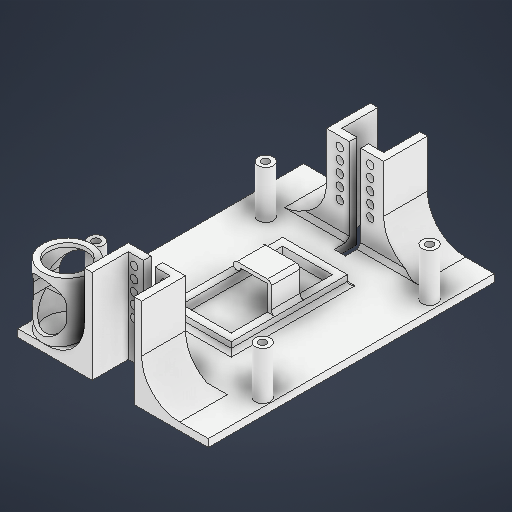
# Autodesk Inventor part: CHASIS
Saved by Autodesk Inventor 2027 (Build 310192060, 192F)
## iProperties
Created: 2026-05-31
Part Number: CHASIS
Material: Genérico
Document SubType Name: Modeling
Designer: noemi
Density: 1 g/cm^3
Appearance: Valor por defecto
Author: noemi
Autodesk Inventor part; units mm, degrees
ref_plane "YZ Plane" through (0, 0, 0) normal (1, 0, 0) x (0, 1, 0)
sketch "Boceto1" plane through (0, 0, 0) normal (0, 1, 0) x (-1, 0, 0)
  line L0 (0, 0) -> (100, 0)
  line L1 (100, 0) -> (100, -150)
  line L2 (100, -150) -> (0, -150)
  line L3 (0, -150) -> (0, 0)
  dimension "d0" = 150
  dimension "d1" = 100
  constraints: 8 end point, 3 perpendicular, 1 horizontal
  measures "d0" distance of L0.end L1.end
  measures "d1" distance of L1.end L2.end
extrude "Extrusión1" add sketch "Boceto1" along normal blind 4
sketch "Boceto2" plane through (0, 4, 0) normal (0, 1, 0) x (1, 0, 0)
  line L0 (-100, 0) -> (0, 0) projected
  line L1 (0, 0) -> (0, 150) projected
  line L2 (-100, 0) -> (0, 0)
  line L3 (-50, 0) -> (-50, 19)
  line L4 (-61, 0) -> (-61, 19)
  line L5 (-39, 0) -> (-39, 19)
  line L6 (-61, 19) -> (-39, 19)
  line L7 (0, 75) -> (-100, 75)
  line L8 (-65, 0) -> (-65, 23)
  line L9 (-65, 23) -> (-35, 23)
  line L10 (-35, 23) -> (-35, 0)
  line L11 (-100, 150) -> (0, 150)
  line L12 (-61, 150) -> (-61, 131)
  line L13 (-39, 150) -> (-39, 131)
  line L14 (-61, 131) -> (-39, 131)
  line L15 (-65, 150) -> (-65, 127)
  line L16 (-65, 127) -> (-35, 127)
  line L17 (-35, 127) -> (-35, 150)
  dimension "d4" = 19
  dimension "d5" = 11
  dimension "d6" = 11
  dimension "d7" = 19
  dimension "d8" = 0
  dimension "d9" = 0
  dimension "d10" = 100
  dimension "d11" = 4
  constraints: 32 end point, 9 symmetric about line, 2 horizontal, 2 midpoint, 2 parallel, 1 perpendicular, 1 vertical, 2 other
  measures "d4" distance of L3.start L3.end
  measures "d5" distance between parallel lines of L3 L4
  measures "d6" distance between parallel lines of L3 L5
  measures "d7" distance between parallel lines of L6 L0
  measures "d8" distance from line of L5.start L0
  measures "d9" distance from line of L4.start L0
  measures "d10" distance from line of L7.end L1
  measures "d11" distance between parallel lines of L4 L8
extrude "Extrusión2" cut sketch "Boceto2" against normal blind 4 contours L4 L6 L3 L0 | L3 L6 L5 L0 | L13 L14 L12 L11
extrude "Extrusión3" add sketch "Boceto2" along normal blind 45 contours L8 L9 L10 L0 L5 L6 L4 | L17 L16 L15 L11 L12 L14 L13
sketch "Boceto3" plane through (-61, 0, -19) normal (0, 0, 1) x (1, 0, 0)
  circle A0 centre (3, 44) radius 2
  line L0 (0, 49) -> (22, 49) projected
  line L1 (11, 49) -> (11, 33.933)
  circle A1 centre (19, 44) radius 2
  point P0 (61, 0)
  dimension "d16" = 4
  dimension "d17" = 8
  dimension "d25" = 5
  constraints: 2 centre point, 2 end point, 1 midpoint, 1 perpendicular, 1 symmetric about line, 1 other
  measures "d16" diameter of A0
  measures "d17" distance from line of L1 A0.centre
  measures "d25" distance from line of L0 A0.centre
extrude "Extrusión4" cut sketch "Boceto3" against normal up to surface (112 mm away)
sketch "Boceto4" plane through (0, 0, 0) normal (0, -1, 0) x (1, 0, 0)
  line L0 (-61, -150) -> (-61, -131) projected
  line L1 (-61, -131) -> (-39, -131) projected
  line L2 (-39, -131) -> (-39, -150) projected
  line L3 (0, -150) -> (-39, -150) projected
  line L4 (0, 0) -> (0, -150) projected
  line L5 (-39, 0) -> (0, 0) projected
  line L6 (-39, 0) -> (-39, -19) projected
  line L7 (-39, -19) -> (-61, -19) projected
  line L8 (-61, -19) -> (-61, 0) projected
  line L9 (-100, 0) -> (-61, 0) projected
  line L10 (-100, -150) -> (-100, 0) projected
  line L11 (-61, -150) -> (-100, -150) projected
  line L12 (-35, -23) -> (-65, -23) projected
  line L13 (-50, -19) -> (-50, -31)
  line L14 (-50, -31) -> (-47, -31)
  line L15 (-47, -31) -> (-47, -19)
  line L16 (-47, -19) -> (-50, -19)
  line L17 (-61, -19) -> (-39, -19) projected
  line L18 (-61, -19) -> (-39, -19)
  line L19 (-50, -31) -> (-53, -31)
  line L20 (-53, -31) -> (-53, -19)
  line L21 (0, -75) -> (-100, -75)
  line L22 (-39, -131) -> (-61, -131)
  line L23 (-50, -119) -> (-47, -119)
  line L24 (-47, -119) -> (-47, -131)
  line L25 (-47, -131) -> (-50, -131)
  line L26 (-50, -119) -> (-53, -119)
  line L27 (-53, -119) -> (-53, -131)
  dimension "d21" = 12
  dimension "d22" = 3
  constraints: 28 end point, 12 symmetric about line, 3 midpoint, 3 point on line, 2 perpendicular, 1 collinear, 1 vertical
  measures "d21" distance of L13.start L13.end
  measures "d22" distance of L13.end L14.end
extrude "Extrusión5" cut sketch "Boceto4" against normal up to surface (49 mm away) contours L27 L26 L23 L24 L1 | L7 L13 L12 L20 | L7 L15 L12 L13 | L12 L13 L19 L20 | L12 L15 L14 L13
fillet "Empalme1" radius 20 4 edges at (-65, 4, -138.5) (-65, 4, -11.5) (-35, 4, -138.5) (-35, 4, -11.5)
sketch "Boceto5" plane through (0, 4, 0) normal (0, 1, 0) x (1, 0, 0)
  circle A0 centre (-86, 116.07) radius 2
  circle A1 centre (-5.3, 121.41) radius 2
  circle A2 centre (-94.3, 35.395) radius 2
  circle A3 centre (-4.51, 33.01) radius 2
  line L0 (0, 0) -> (0, 150) projected
  line L1 (-65, 150) -> (-85, 150) projected
  line L2 (-5.3, 86.5785) -> (-5.3, 135.0177)
  line L3 (-100, 150) -> (-100, 0) projected
  line L4 (0, 150) -> (-15, 150) projected
  line L5 (-4.51, 30.5987) -> (-4.51, 75)
  circle A4 centre (-86, 116.07) radius 4
  circle A5 centre (-5.3, 121.41) radius 4
  circle A6 centre (-94.3, 35.395) radius 4
  circle A7 centre (-4.51, 33.01) radius 4
  dimension "d27" = 4
  dimension "d28" = 4
  dimension "d29" = 4
  dimension "d30" = 4
  dimension "d32" = 33.93
  dimension "d33" = 80.7
  dimension "d34" = 14
  dimension "d35" = 28.59
  dimension "d36" = 114.605
  dimension "d37" = 5.7
  dimension "d38" = 81.49
  dimension "d39" = 88.4
  dimension "d40" = 2
  dimension "d41" = 2
  dimension "d42" = 2
  dimension "d43" = 2
  dimension "d54" = 80.675
  constraints: 8 centre point, 4 end point, 2 point on line, 2 vertical
  measures "d27" diameter of A0
  measures "d28" diameter of A1
  measures "d29" diameter of A2
  measures "d30" diameter of A3
  measures "d32" distance from line of L1 A0.centre
  measures "d33" distance from line of L2 A0.centre
  measures "d34" distance from line of L3 A0.centre
  measures "d35" distance from line of L4 A1.centre
  measures "d36" distance from line of L1 A2.centre
  measures "d37" distance from line of L3 A2.centre
  measures "d38" distance from line of L5 A0.centre
  measures "d39" vertical distance of A3.centre A1.centre
  measures "d40" radial gap between concentric circles of A0 A4
  measures "d41" radial gap between concentric circles of A1 A5
  measures "d42" radial gap between concentric circles of A2 A6
  measures "d43" radial gap between concentric circles of A3 A7
  measures "d54" vertical distance of A2.centre A0.centre
extrude "Extrusión6" add sketch "Boceto5" along normal blind 25 contours A1 L2 A5 | A1 L2 A5 | A7 | A4 | A6
thread "Rosca1" size "M4x0.7" class "6H" standard "ISO Metric profile" full length
thread "Rosca2" size "M4x0.7" class "6H" standard "ISO Metric profile" full length
thread "Rosca3" size "M4x0.7" class "6H" standard "ISO Metric profile" full length
thread "Rosca4" size "M4x0.7" class "6H" standard "ISO Metric profile" full length
sketch "Boceto6" plane through (0, 4, 0) normal (0, 1, 0) x (1, 0, 0)
  line L0 (-63, 49) -> (-37, 49)
  line L1 (-37, 49) -> (-37, 102)
  line L2 (-37, 102) -> (-63, 102)
  line L3 (-63, 102) -> (-63, 49)
  line L4 (-33, 45) -> (-67, 45)
  line L5 (-67, 45) -> (-67, 106)
  line L6 (-67, 106) -> (-33, 106)
  line L7 (-33, 106) -> (-33, 45)
  line L8 (-100, 150) -> (-100, 0) projected
  line L9 (0, 150) -> (-15, 150) projected
  line L10 (0, 0) -> (0, 150) projected
  dimension "d55" = 53
  dimension "d56" = 26
  dimension "d57" = 4
  dimension "d58" = 33
  dimension "d59" = 44
  dimension "d93" = 33
  constraints: 16 end point, 6 perpendicular, 1 horizontal, 3 other
  measures "d55" distance of L0.end L1.end
  measures "d56" distance of L0.start L0.end
  measures "d57" distance between parallel lines of L0 L4
  measures "d58" distance between parallel lines of L8 L5
  measures "d59" distance between parallel lines of L9 L6
  measures "d93" distance between parallel lines of L10 L7
extrude "Extrusión7" add sketch "Boceto6" along normal blind 5
ref_plane "Plano de trabajo1" through (-67, 4, -75.5) normal (0, 0, 1) x (1, 0, 0)
sketch "Boceto7" plane through (-67, 4, -75.5) normal (0, 0, 1) x (1, 0, 0)
  line L0 (14, 20) -> (28, 20)
  line L1 (52, 0) -> (20, 0) projected
  line L2 (34, 0) -> (34, 5) projected
  line L3 (34, 5) -> (34, 20)
  line L4 (14, 0) -> (14, 45) projected
  line L5 (14, 20) -> (14, 18)
  line L6 (-3.7901, 18) -> (30, 18)
  line L7 (30, 5) -> (30, 18)
  line L8 (32, 5) -> (32, 18)
  line L9 (30, 20) -> (-3.7901, 20)
  arc A0 (32, 18) -> (30, 20) centre (30, 18) ccw
  line L10 (30, 0) -> (30, 5) projected
  line L11 (30, 5) -> (32, 5)
  line L12 (34, 5) -> (0, 5) projected
  circle A1 centre (14, 18) radius 2
  point P0 (67, -4)
  point P1 (14, 18)
  dimension "d64" = 2
  dimension "d65" = 2
  dimension "d66" = 2
  dimension "d67" = 2
  dimension "d72" = 18
  constraints: 16 end point, 3 point on line, 2 horizontal, 2 point on circle, 2 tangent, 1 centre point, 1 coincident, 1 collinear, 1 perpendicular, 1 vertical, 1 vertical alignment, 3 other
  measures "d64" distance of L0.start L5.end
  measures "d65" distance between parallel lines of L0 L6
  measures "d66" distance between parallel lines of L7 L8
  measures "d67" radius of A0
  measures "d72" distance between parallel lines of L1 L6
extrude "Extrusión8" add sketch "Boceto7" along normal mid plane 15 contours A1 L6 L4 | L0 L9 A0 L8 L11 L7 L6 A1 picked at (14.4376, 19.2506)
extrude "Extrusión9" cut sketch "Boceto5" against normal blind 30 contours A0 | A1 L2 | L2 A1 | A2 | A3 L5 | L5 A3
extrude "Extrusión10" add sketch "Boceto7" along normal mid plane 15 contours A1 L6 L4 | L4 L6 A1 | L6 A1 L4 | L4 A1 L6
fillet "Empalme2" radius 2 4 edges at (-33, 4, -75.5) (-50, 4, -45) (-50, 4, -106) (-67, 4, -75.5)
fillet "Empalme3" radius 2 1 edges at (-35, 9, -75.5)
chamfer "Chaflán1" distance 2 angle 45 4 edges at (-69, 4, -127) (-31, 4, -127) (-31, 4, -23) (-69, 4, -23)
sketch "Boceto8" plane through (0, 4, 0) normal (0, 1, 0) x (1, 0, 0)
  circle A0 centre (-107.7943, -40.3526) radius 10
  circle A1 centre (-107.7943, -40.3526) radius 13
  circle A2 centre (-87, 13) radius 13
  line L0 (-47, 119) -> (-47, 131) projected
  line L1 (-47, 131) -> (-39, 131) projected
  line L2 (-39, 131) -> (-39, 150) projected
  line L3 (0, 150) -> (-39, 150) projected
  line L4 (0, 0) -> (0, 150) projected
  line L5 (-39, 0) -> (0, 0) projected
  line L6 (-39, 0) -> (-39, 19) projected
  line L7 (-39, 19) -> (-47, 19) projected
  line L8 (-47, 19) -> (-47, 31) projected
  line L9 (-47, 31) -> (-53, 31) projected
  line L10 (-53, 31) -> (-53, 19) projected
  line L11 (-53, 19) -> (-61, 19) projected
  line L12 (-61, 19) -> (-61, 0) projected
  line L13 (-100, 0) -> (-61, 0) projected
  line L14 (-100, 150) -> (-100, 0) projected
  line L15 (-61, 150) -> (-100, 150) projected
  line L16 (-61, 150) -> (-61, 131) projected
  line L17 (-61, 131) -> (-53, 131) projected
  line L18 (-53, 131) -> (-53, 119) projected
  line L19 (-53, 119) -> (-47, 119) projected
  circle A3 centre (-87, 13) radius 11
  dimension "d80" = 20
  dimension "d81" = 3
  dimension "d82" = 26
  dimension "d83" = 2
  constraints: 4 centre point, 2 tangent
  measures "d80" diameter of A0
  measures "d81" radial gap between concentric circles of A0 A1
  measures "d82" diameter of A2
  measures "d83" radial gap between concentric circles of A2 A3
extrude "Extrusión11" add sketch "Boceto8" along normal blind 30 contours A2
sketch "Boceto9" plane through (-87, 34, -13) normal (0, 1, 0) x (1, 0, 0)
  circle A0 centre (0, 0) radius 10
  circle A1 centre (0, 0) radius 13 projected
  point P0 (87, -13)
  dimension "d86" = 20
  constraints: 1 centre point
  measures "d86" diameter of A0
extrude "Extrusión12" add sketch "Boceto9" along normal blind 2
ref_plane "Plano de trabajo2" through (-100, 4, 0) normal (0, 0, 1) x (1, 0, 0)
sketch "Boceto10" plane through (-100, 4, 0) normal (0, 0, 1) x (1, 0, 0)
  line L0 (12, 25) -> (12, -4) projected
  circle A0 centre (12, 13.2071) radius 10
  circle A1 centre (12, 19.1516) radius 10
  line L1 (22, 19.1516) -> (22, 13.2071)
  line L2 (1.7, 0) -> (1.7, 25) projected
  line L3 (2, 25.8487) -> (2, 7.4902)
  point P0 (100, -4)
  point P1 (2, 19.1516)
  point P2 (2, 13.2071)
  dimension "d91" = 20
  dimension "d92" = 20
  constraints: 4 end point, 3 vertical, 2 point on line, 1 parallel, 6 other
extrude "Extrusión13" cut sketch "Boceto10" against normal blind 30
pattern_linear "Patrón rectangular1" count 5 spacing 6 along (0, -1, 0) of "Extrusión4"
